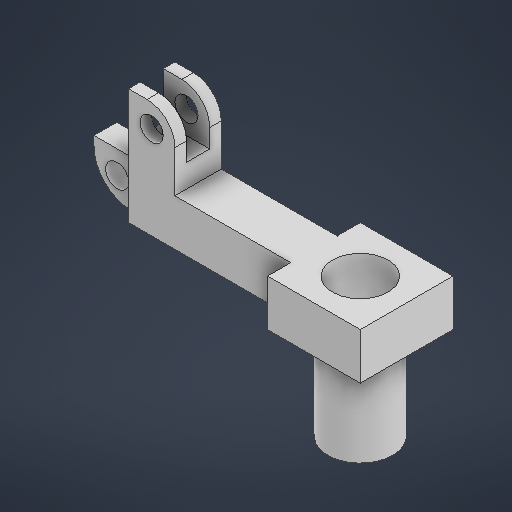
# Autodesk Inventor part: Press_Lower_Arm
Saved by Autodesk Inventor 2026.1 (Build 301233020, 233B)
## iProperties
Created: 2025-09-29
Part Number: Press_Lower_Arm
Material: Generic
Document SubType Name: Modeling
Designer: Gamec
Density: 1 g/cm^3
Appearance: Default
Author: Gamec
Autodesk Inventor part; units mm, degrees
ref_plane "YZ Plane" through (0, 0, 0) normal (1, 0, 0) x (0, 1, 0)
ref_plane "XZ Plane" through (0, 0, 0) normal (0, 1, 0) x (-1, 0, 0)
ref_plane "XY Plane" through (0, 0, 0) normal (0, 0, 1) x (1, 0, 0)
sketch "Sketch1" plane through (0, 0, 0) normal (0, 1, 0) x (-1, 0, 0)
  line L0 (-34.925, 6.35) -> (34.925, 6.35)
  line L1 (34.925, 6.35) -> (34.925, -6.35)
  line L2 (34.925, -6.35) -> (-34.925, -6.35)
  line L3 (-34.925, -6.35) -> (-34.925, 6.35)
  line L4 (-34.925, 6.35) -> (34.925, -6.35) construction
  line L5 (34.925, 6.35) -> (-34.925, -6.35) construction
  point P0 (0, 0)
  dimension "d0" = 69.85
  dimension "d1" = 12.7
  constraints: 12 end point, 2 midpoint, 2 parallel, 1 horizontal, 1 perpendicular
  measures "d0" distance of L1.end L2.end
  measures "d1" distance of L0.end L1.end
extrude "Extrusion1" add sketch "Sketch1" along normal blind 12.7
sketch "Sketch2" plane through (-34.925, 0, -6.35) normal (-1, 0, 0) x (0, 0, 1)
  line L0 (0, 12.7) -> (12.7, 12.7) projected
  line L1 (3.2385, 0) -> (9.4615, 0)
  line L2 (9.4615, 0) -> (9.4615, 12.7)
  line L3 (9.4615, 12.7) -> (3.2385, 12.7)
  line L4 (3.2385, 12.7) -> (3.2385, 0)
  line L5 (3.2385, 0) -> (9.4615, 12.7) construction
  line L6 (9.4615, 0) -> (3.2385, 12.7) construction
  line L7 (12.7, 0) -> (12.7, 12.7) projected
  point P0 (6.35, 0)
  point P1 (6.35, 6.35)
  dimension "d4" = 6.223
  dimension "d5" = 12.7
  dimension "d6" = 3.2385
  constraints: 12 end point, 2 midpoint, 2 parallel, 1 horizontal, 1 perpendicular, 1 point on line
  measures "d4" distance of L3.end L2.end
  measures "d5" distance of L1.end L2.end
  measures "d6" distance between parallel lines of L7 L2
extrude "Extrusion2" add sketch "Sketch2" along normal blind 12.7
fillet "Fillet1" radius 10.16 1 edges at (-47.625, 0, 0)
sketch "Sketch3" plane through (-34.925, 0, 3.1115) normal (0, 0, 1) x (1, 0, 0)
  circle A0 centre (-6.35, 6.35) radius 3.175
  line L0 (0, 12.7) -> (-12.7, 12.7) projected
  line L1 (-12.7, 10.16) -> (-12.7, 12.7) projected
  point P0 (34.925, 0)
  dimension "d10" = 6.35
  dimension "d41" = 6.35
  dimension "d42" = 6.35
  constraints: 1 centre point
  measures "d10" diameter of A0
  measures "d41" distance from line of L0 A0.centre
  measures "d42" distance from line of L1 A0.centre
extrude "Extrusion3" cut sketch "Sketch3" against normal blind 12.7
sketch "Sketch4" plane through (0, 12.7, 0) normal (0, 1, 0) x (1, 0, 0)
  line L0 (-34.925, -3.1115) -> (-34.925, -6.35) projected
  line L1 (34.925, 6.35) -> (-34.925, 6.35) projected
  line L2 (-34.925, -6.35) -> (-22.225, -6.35)
  line L3 (-22.225, -6.35) -> (-22.225, 6.35)
  line L4 (-22.225, 6.35) -> (-34.925, 6.35)
  line L5 (-34.925, 6.35) -> (-34.925, -6.35)
  point P0 (0, 0)
  point P1 (-34.925, 6.35)
  dimension "d13" = 12.7
  constraints: 8 end point, 2 parallel, 1 horizontal, 1 perpendicular, 1 point on line
  measures "d13" distance of L4.end L3.end
extrude "Extrusion4" add sketch "Sketch4" along normal blind 19.05
sketch "Sketch5" plane through (0, 31.75, 0) normal (0, 1, 0) x (1, 0, 0)
  line L0 (-34.925, -3.1115) -> (-34.925, -6.35) projected
  line L1 (-22.225, -6.35) -> (-22.225, 6.35) projected
  line L2 (-34.925, -3.175) -> (-22.225, -3.175)
  line L3 (-22.225, -3.175) -> (-22.225, 3.175)
  line L4 (-22.225, 3.175) -> (-34.925, 3.175)
  line L5 (-34.925, 3.175) -> (-34.925, -3.175)
  line L6 (-34.925, -6.35) -> (-22.225, -6.35) projected
  point P0 (0, 0)
  point P1 (-28.575, -6.35)
  dimension "d16" = 6.35
  dimension "d17" = 3.175
  constraints: 8 end point, 2 parallel, 2 point on line, 1 horizontal, 1 midpoint, 1 perpendicular
  measures "d16" distance of L3.end L2.end
  measures "d17" distance from line of point (-28.575, -6.35) L2
extrude "Extrusion5" cut sketch "Sketch5" against normal blind 12.7 contours L5 L4 L1 L2 L0
sketch "Sketch6" plane through (-34.925, 0, 6.35) normal (0, 0, 1) x (1, 0, 0)
  circle A0 centre (6.35, 25.4) radius 3.175
  line L0 (0, 31.75) -> (12.7, 31.75) projected
  line L1 (0, 0) -> (0, 31.75) projected
  point P0 (34.925, 0)
  dimension "d20" = 6.35
  dimension "d21" = 6.35
  dimension "d43" = 6.35
  constraints: 1 centre point
  measures "d20" diameter of A0
  measures "d21" distance from line of L0 A0.centre
  measures "d43" distance from line of L1 A0.centre
extrude "Extrusion6" cut sketch "Sketch6" against normal blind 12.7
sketch "Sketch7" plane through (0, 12.7, 0) normal (0, 1, 0) x (1, 0, 0)
  line L0 (34.925, -12.7) -> (9.525, -12.7)
  line L1 (9.525, -12.7) -> (9.525, 12.7)
  line L2 (9.525, 12.7) -> (34.925, 12.7)
  line L3 (34.925, 12.7) -> (34.925, -12.7)
  line L4 (34.925, -6.35) -> (34.925, 6.35) projected
  line L5 (-22.225, -6.35) -> (34.925, -6.35) projected
  point P0 (0, 0)
  dimension "d24" = 25.4
  dimension "d25" = 25.4
  dimension "d26" = 25.4
  dimension "d27" = 6.35
  constraints: 8 end point, 2 parallel, 1 horizontal, 1 perpendicular
  measures "d24" distance of L2.end L0.start
  measures "d25" distance between parallel lines of L4 L1
  measures "d26" distance of L1.end L2.end
  measures "d27" distance between parallel lines of L5 L0
extrude "Extrusion7" add sketch "Sketch7" against normal blind 12.7
sketch "Sketch8" plane through (0, 0, 0) normal (0, -1, 0) x (1, 0, 0)
  circle A0 centre (22.225, 0) radius 8.89
  circle A1 centre (22.225, 0) radius 7.62
  line L0 (34.925, 12.7) -> (34.925, -12.7) projected
  point P0 (0, 0)
  dimension "d30" = 17.78
  dimension "d31" = 15.24
  dimension "d39" = 12.7
  constraints: 2 centre point, 1 coincident
  measures "d30" diameter of A0
  measures "d31" diameter of A1
  measures "d39" distance from line of L0 A0.centre
extrude "Extrusion8" add sketch "Sketch8" along normal blind 25.4
sketch "Sketch9" plane through (22.225, -25.4, 0) normal (0, -1, 0) x (1, 0, 0)
  circle A0 centre (0, 0) radius 6.3
  circle A1 centre (0, 0) radius 7.62
  point P0 (-22.225, 0)
  dimension "d34" = 12.6
  constraints: 2 centre point, 1 coincident
  measures "d34" diameter of A0
extrude "Extrusion9" add sketch "Sketch9" against normal blind 2.54
sketch "Sketch10" plane through (22.225, 0, 0) normal (0, -1, 0) x (1, 0, 0)
  circle A0 centre (0, 0) radius 7.62
  point P0 (-22.225, 0)
  constraints: 1 centre point
extrude "Extrusion10" cut sketch "Sketch10" against normal blind 25.4
fillet "Fillet2" radius 7.62 2 edges at (-22.225, 31.75, 4.7625) (-22.225, 31.75, -4.7625)
body "Solid1"
